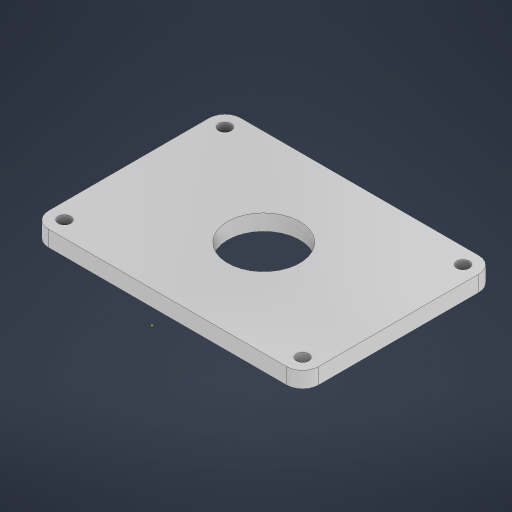
# Autodesk Inventor part: Top Plate
Saved by Autodesk Inventor 2024.3 (Build 283343000, 343)
## iProperties
Created: 2024-07-07
Part Number: Top Plate
Material: Aluminum 6061
Document SubType Name: Modeling
Designer: kaito
Density: 2.7 g/cm^3
Appearance: Aluminum - Polished
Author: kaito
Autodesk Inventor part; units mm, degrees
ref_plane "YZ Plane" through (0, 0, 0) normal (1, 0, 0) x (0, 1, 0)
ref_plane "XZ Plane" through (0, 0, 0) normal (0, 1, 0) x (-1, 0, 0)
ref_plane "XY Plane" through (0, 0, 0) normal (0, 0, 1) x (1, 0, 0)
sketch "Sketch1" plane through (0, 0, 0) normal (0, 1, 0) x (-1, 0, 0)
  point P0 (0, 0)
sketch "Sketch2" plane through (0, 0, 0) normal (0, 1, 0) x (-1, 0, 0)
  circle A0 centre (0, 0) radius 6.35 construction
  circle A1 centre (0, -44.45) radius 38.1 construction
  circle A2 centre (0, 0) radius 25.4 construction
  circle A3 centre (17.9605, -17.9605) radius 2.4892 construction
  circle A4 centre (25.4, 0) radius 2.4892 construction
  circle A5 centre (17.9605, 17.9605) radius 2.4892 construction
  circle A6 centre (0, 25.4) radius 2.4892 construction
  circle A7 centre (-17.9605, 17.9605) radius 2.4892 construction
  circle A8 centre (-25.4, 0) radius 2.4892 construction
  circle A9 centre (-17.9605, -17.9605) radius 2.4892 construction
  circle A10 centre (0, -25.4) radius 2.4892 construction
  circle A11 centre (0, -88.9) radius 25.4 construction
  circle A12 centre (0, -88.9) radius 6.35 construction
  circle A13 centre (-17.9605, -70.9395) radius 2.4892 construction
  circle A14 centre (-25.4, -88.9) radius 2.4892 construction
  circle A15 centre (-17.9605, -106.8605) radius 2.4892 construction
  circle A16 centre (0, -114.3) radius 2.4892 construction
  circle A17 centre (17.9605, -106.8605) radius 2.4892 construction
  circle A18 centre (25.4, -88.9) radius 2.4892 construction
  circle A19 centre (17.9605, -70.9395) radius 2.4892 construction
  circle A20 centre (0, -63.5) radius 2.4892 construction
  circle A21 centre (0, 0) radius 9.525 construction
  circle A22 centre (0, -88.9) radius 9.525 construction
  circle A23 centre (47.3968, -12.5178) radius 6.35 construction
  circle A24 centre (47.3968, -76.3822) radius 6.35 construction
  circle A25 centre (-47.3968, -76.3822) radius 6.35 construction
  circle A26 centre (0, 0) radius 29.972 construction
  circle A27 centre (0, -88.9) radius 29.972 construction
  circle A28 centre (-47.3968, -12.5178) radius 6.35 construction
  circle A29 centre (47.3968, -12.5178) radius 2.4892
  circle A30 centre (47.3968, -76.3822) radius 2.4892
  circle A31 centre (-47.3968, -12.5178) radius 2.4892
  circle A32 centre (-47.3968, -76.3822) radius 2.4892
  line L0 (42.1305, -72.8341) -> (31.5979, -65.7381) construction
  line L1 (41.2573, -78.0036) -> (28.9784, -81.2466) construction
  line L2 (-41.2573, -78.0036) -> (-28.9784, -81.2466) construction
  line L3 (-42.1305, -72.8341) -> (-31.5979, -65.7381) construction
  line L4 (-41.2573, -10.8964) -> (-28.9784, -7.6534) construction
  line L5 (-42.1305, -16.0659) -> (-31.5979, -23.1619) construction
  line L6 (41.2573, -10.8964) -> (28.9784, -7.6534) construction
  line L7 (42.1305, -16.0659) -> (31.5979, -23.1619) construction
  circle A33 centre (0, -44.45) radius 14.351
  line L8 (47.3968, -82.7322) -> (-47.3968, -82.7322)
  line L9 (-53.7468, -76.3822) -> (-53.7468, -12.5178)
  line L10 (-47.3968, -6.1678) -> (47.3968, -6.1678)
  line L11 (53.7468, -12.5178) -> (53.7468, -76.3822)
  arc A34 (53.7468, -12.5178) -> (47.3968, -6.1678) centre (47.3968, -12.5178) ccw
  arc A35 (-53.7468, -76.3822) -> (-47.3968, -82.7322) centre (-47.3968, -76.3822) ccw
  arc A36 (-47.3968, -6.1678) -> (-53.7468, -12.5178) centre (-47.3968, -12.5178) ccw
  arc A37 (47.3968, -82.7322) -> (53.7468, -76.3822) centre (47.3968, -76.3822) ccw
  point P0 (-20.6699, 21.7043)
  point P1 (-20.6699, -110.6043)
  point P2 (51.7761, -80.9805)
  point P3 (51.7761, -7.9195)
  point P4 (-47.3968, -82.7322)
  dimension "d2" = 50.8
  dimension "d0" = 12.7
  dimension "d1" = 76.2
  dimension "d3" = 4.9784
  dimension "d6" = 360
  dimension "d8" = 4.9784
  dimension "d11" = 360
  dimension "d13" = 19.05
  dimension "d14" = 19.05
  dimension "d15" = 59.944
  dimension "d16" = 59.944
  dimension "d17" = 12.7
  dimension "d18" = 4.9784
  dimension "d24" = 12.7
  dimension "d25" = 28.702
  constraints: 41 point on circle, 36 centre point, 24 end point, 16 point on line, 13 tangent, 12 coincident, 8 equal radius, 7 equal length, 4 vertical alignment, 2 perpendicular, 40 other
  measures "d0" diameter of A0
  measures "d1" diameter of A1
  measures "d3" diameter of A3
  measures "d8" diameter of A13
  measures "d13" diameter of A21
  measures "d14" diameter of A22
  measures "d15" diameter of A26
  measures "d16" diameter of A27
  measures "d17" diameter of A23
  measures "d18" diameter of A29
  measures "d24" distance of L0.start L0.end
  measures "d25" diameter of A33
extrude "Extrusion2" add sketch "Sketch2" along normal blind 6.35
body "Solid2"
